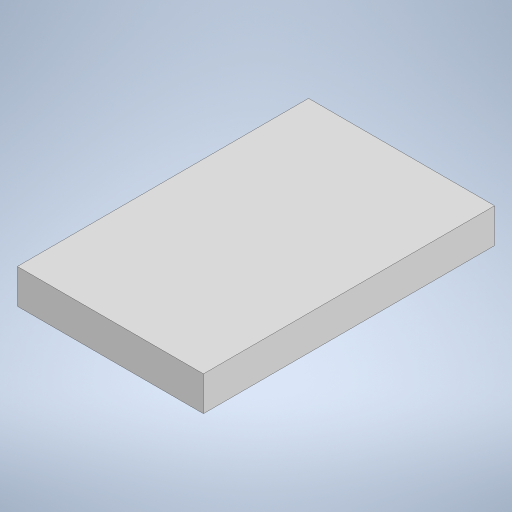
# Autodesk Inventor part: 麵包板
Saved by Autodesk Inventor 2024 (Build 280153000, 153)
## iProperties
Created: 2024-04-10
Part Number: 麵包板
Material: 一般
Document SubType Name: Modeling
Designer: rumse
Density: 1 g/cm^3
Appearance: 預設
Author: rumse
Autodesk Inventor part; units mm, degrees
ref_plane "YZ Plane" through (0, 0, 0) normal (1, 0, 0) x (0, 1, 0)
ref_plane "XZ Plane" through (0, 0, 0) normal (0, 1, 0) x (-1, 0, 0)
ref_plane "XY Plane" through (0, 0, 0) normal (0, 0, 1) x (1, 0, 0)
sketch "草圖1" plane through (0, 0, 0) normal (0, 1, 0) x (-1, 0, 0)
  line L0 (0, 0) -> (54, 0)
  line L1 (54, 0) -> (54, -84.5)
  line L2 (54, -84.5) -> (0, -84.5)
  line L3 (0, -84.5) -> (0, 0)
  dimension "d0" = 54
  dimension "d1" = 84.5
  constraints: 8 end point, 2 parallel, 1 horizontal, 1 perpendicular
  measures "d0" distance of L1.end L2.end
  measures "d1" distance of L0.end L1.end
extrude "擠出1" add sketch "草圖1" along normal blind 10
